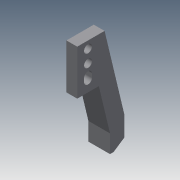
# Autodesk Inventor part: HbBatteryDoorLever03
Saved by Autodesk Inventor 2015 SP1 (Build 190203100, 203)
## iProperties
Created: 2015-04-03
Part Number: HbBatteryDoorLever03
Material: 一般
Document SubType Name: Modeling
Designer: Yamaura
Density: 1 g/cm^3
Appearance: 既定
Author: Yamaura
Autodesk Inventor part; units mm, degrees
ref_plane "YZ Plane" through (0, 0, 0) normal (1, 0, 0) x (0, 1, 0)
ref_plane "XZ Plane" through (0, 0, 0) normal (0, 1, 0) x (-1, 0, 0)
ref_plane "XY Plane" through (0, 0, 0) normal (0, 0, 1) x (1, 0, 0)
sketch "スケッチ1" plane through (0, 0, 0) normal (1, 0, 0) x (0, 1, 0)
  circle A0 centre (0, 0) radius 1.1
  circle A1 centre (0, -3.5) radius 1.1
  circle A2 centre (0, 3.5) radius 1.1
  circle A3 centre (0, -3) radius 1.1
  circle A4 centre (0, -4) radius 1.1
  line L0 (1.1, -3) -> (1.1, -4)
  line L1 (-1.1, -3) -> (-1.1, -4)
  line L2 (3, 5.5) -> (-3, 5.5)
  line L3 (-3, 5.5) -> (-3, -7)
  line L4 (-3, -7) -> (3, -7)
  line L5 (3, -7) -> (3, 5.5)
  dimension "d0" = 2.2
  dimension "d1" = 2.2
  dimension "d2" = 2.2
  dimension "d3" = 3.5
  dimension "d4" = 3.5
  dimension "d5" = 2.2
  dimension "d6" = 2.2
  dimension "d7" = 0.5
  dimension "d8" = 0.5
  dimension "d9" = 3
  dimension "d10" = 6
  dimension "d11" = 5.5
  dimension "d12" = 12.5
  constraints: 12 end point, 5 centre point, 4 point on circle, 2 parallel, 2 tangent, 2 vertical, 1 coincident, 1 horizontal, 1 perpendicular
  measures "d0" diameter of A0
  measures "d1" diameter of A1
  measures "d2" diameter of A2
  measures "d3" distance of point (0, 0) A2.centre
  measures "d4" distance of A1.centre point (0, 0)
  measures "d5" diameter of A3
  measures "d6" diameter of A4
  measures "d7" distance of A1.centre A3.centre
  measures "d8" distance of A4.centre A1.centre
  measures "d9" distance from line of L5 point (0, 0)
  measures "d10" distance of L3.end L4.end
  measures "d11" distance from line of L2 point (0, 0)
  measures "d12" distance of L2.end L3.end
extrude "押し出し1" add sketch "スケッチ1" against normal blind 3
sketch "スケッチ3" plane through (0, 0, 0) normal (1, 0, 0) x (0, 1, 0)
  circle A0 centre (0, 3.5) radius 1.1 projected
  circle A1 centre (0, 0) radius 1.1 projected
  arc A2 (-1.1, -3) -> (1.1, -3) centre (0, -3) ccw projected
  line L0 (1.1, -3) -> (1.1, -4) projected
  arc A3 (1.1, -4) -> (-1.1, -4) centre (0, -4) ccw projected
  line L1 (-1.1, -4) -> (-1.1, -3) projected
  line L2 (-3, -7) -> (3, -7)
  line L3 (3, 5.5) -> (4.6, 5.5)
  line L4 (4.6, 5.5) -> (10.1, -17.3871)
  line L5 (10.1, -17.3871) -> (10.1, -24.8935)
  line L6 (10.1, -24.8935) -> (6.1, -24.8935)
  line L7 (6.1, -24.8935) -> (6.1, -19.9)
  line L8 (6.1, -19.9) -> (3, -7)
  line L9 (3, 5.5) -> (3, -7)
  dimension "d19" = 1.6
  dimension "d34" = 4
  dimension "d35" = 12.9
  dimension "d38" = 3.1
  constraints: 16 end point, 4 centre point, 2 perpendicular, 2 vertical, 1 parallel, 1 point on line
  measures "d19" distance of L3.start L3.end
  measures "d34" distance of L5.end L6.end
  measures "d35" vertical distance of L7.end L8.end
  measures "d38" horizontal distance of L7.end L8.end
extrude "押し出し4" add sketch "スケッチ3" against normal blind 3 contours L3 L4 L5 L6 L7 L8 L9
chamfer "面取り1" distance 2 distance2 3 1 edges at (-1.5, 10.1, -24.8935) measured on face at (-1.5, 10.1, -24.3935)
sketch "スケッチ4" plane through (-3, 0, 0) normal (-1, 0, 0) x (0, 0, 1)
  line L0 (-24.8935, 7.1) -> (-22.8935, 10.1)
  line L1 (-24.8935, 7.1) -> (-24.8935, 6.1)
  line L2 (-24.8935, 6.1) -> (-19.9, 6.1)
  line L3 (-19.9, 6.1) -> (-7, 3)
  line L4 (-7, 3) -> (-7, -3) projected
  line L5 (-7, -3) -> (5.5, -3) projected
  line L6 (5.5, -3) -> (5.5, 4.6) projected
  line L7 (-5.954, 7.3525) -> (-17.3871, 10.1)
  line L8 (-17.3871, 10.1) -> (-22.8935, 10.1)
  circle A0 centre (3.5, 0) radius 1.1 projected
  circle A1 centre (0, 0) radius 1.1 projected
  arc A2 (-3, 1.1) -> (-3, -1.1) centre (-3, 0) ccw projected
  line L9 (-3, -1.1) -> (-4, -1.1) projected
  arc A3 (-4, -1.1) -> (-4, 1.1) centre (-4, 0) ccw projected
  line L10 (-4, 1.1) -> (-3, 1.1) projected
  line L11 (5.5, 4.6) -> (-17.3871, 10.1) projected
  line L12 (-7, 3) -> (-5.954, 7.3525)
  constraints: 14 end point, 4 centre point, 1 perpendicular, 1 point on line
extrude "押し出し5" add sketch "スケッチ4" along normal blind 3 contours L0 L8 L7 L12 L3 L2 L1
chamfer "面取り2" distance 3 distance2 3 1 edges at (-6, 5.1763, -6.477) measured on face at (-6, 5.2931, -6.9632)
